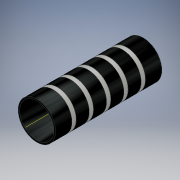
# Autodesk Inventor part: MIddle Rod Cover
Saved by Autodesk Inventor 2018 (Build 220112000, 112)
## iProperties
Created: 2018-02-14
Part Number: MIddle Rod Cover
Material: Stainless Steel
Document SubType Name: Modeling
Designer: Cole
Density: 8 g/cm^3
Appearance: Gunmetal - Polished
Author: Cole
Autodesk Inventor part; units mm, degrees
ref_plane "YZ Plane" through (0, 0, 0) normal (1, 0, 0) x (0, 1, 0)
ref_plane "XZ Plane" through (0, 0, 0) normal (0, 1, 0) x (-1, 0, 0)
ref_plane "XY Plane" through (0, 0, 0) normal (0, 0, 1) x (1, 0, 0)
sketch "Sketch1" plane through (0, 0, 0) normal (0, 0, 1) x (1, 0, 0)
  circle A0 centre (0, 0) radius 17.4625
  dimension "d0" = 34.925
  constraints: 1 centre point, 1 coincident
  measures "d0" diameter of A0
extrude "Extrusion1" add sketch "Sketch1" along normal mid plane 99.06
sketch "Sketch2" plane through (0, 0, 49.53) normal (0, 0, 1) x (1, 0, 0)
  circle A0 centre (0, 0) radius 15.9385
  circle A1 centre (0, 0) radius 17.4625 projected
  dimension "d16" = 1.524
  constraints: 1 centre point, 1 coincident
  measures "d16" radial gap between concentric circles of A0 A1
extrude "Extrusion2" cut sketch "Sketch2" against normal blind 99.06 contours A0
sketch "Sketch3" plane through (0, 0, 0) normal (0, 0, 1) x (1, 0, 0)
  circle A0 centre (0, 0) radius 17.3355
  circle A1 centre (0, 0) radius 17.4625
  dimension "d6" = 34.671
  constraints: 2 centre point, 2 coincident
  measures "d6" diameter of A0
extrude "Extrusion3" cut sketch "Sketch3" along normal mid plane 3.9688
pattern_linear "Rectangular Pattern1" count 3 spacing 16.129 along (0, 0, 1) count 3 spacing 16.129 along (0, 0, -1) of "Extrusion3"
body "Solid1"
